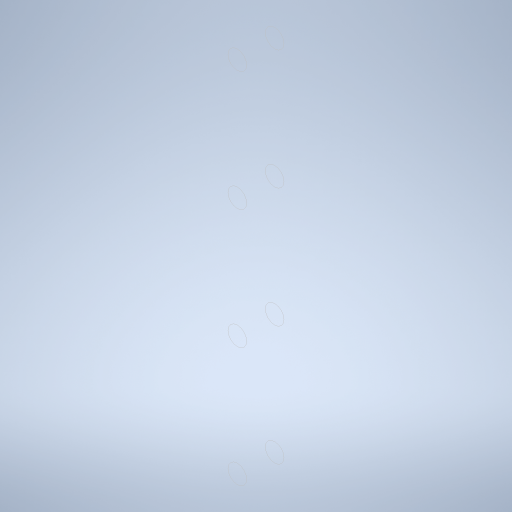
# Autodesk Inventor part: front_holes
Saved by Autodesk Inventor 2024 (Build 280153000, 153)
## iProperties
Created: 2019-12-13
Part Number: front_holes
Material: Generic
Document SubType Name: Modeling
Designer: RokasM
Density: 1 g/cm^3
Appearance: Default
Author: RokasM
Autodesk Inventor part; units mm, degrees
ref_plane "YZ Plane" through (0, 0, 0) normal (1, 0, 0) x (0, 1, 0)
ref_plane "XZ Plane" through (0, 0, 0) normal (0, 1, 0) x (-1, 0, 0)
ref_plane "XY Plane" through (0, 0, 0) normal (0, 0, 1) x (1, 0, 0)
sketch "Sketch1" plane through (0, 0, 0) normal (0, 1, 0) x (-1, 0, 0)
  circle A0 centre (0, 48) radius 2.5
  circle A1 centre (0, 16) radius 2.5
  circle A2 centre (0, -16) radius 2.5
  circle A3 centre (0, -48) radius 2.5
  point P0 (0, 0)
  dimension "d0" = 5
  dimension "d1" = 5
  dimension "d2" = 5
  dimension "d3" = 5
  dimension "d4" = 32
  dimension "d5" = 32
  dimension "d6" = 32
  dimension "d7" = 16
  constraints: 4 centre point, 4 vertical alignment
  measures "d0" diameter of A0
  measures "d1" diameter of A1
  measures "d2" diameter of A2
  measures "d3" diameter of A3
  measures "d4" distance of A1.centre A0.centre
  measures "d5" distance of A2.centre A1.centre
  measures "d6" distance of A2.centre A3.centre
  measures "d7" distance of point (0, 0) A2.centre
extrude "Extrusion1" add sketch "Sketch1" against normal blind 10
